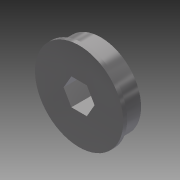
# Autodesk Inventor part: Hex Bearing 3-8 in (FR6ZZL-hex (am-0692))
Saved by Autodesk Inventor 2014 (Build 180170000, 170)
## iProperties
Created: 2014-01-12
Part Number: Hex Bearing 3-8 in (FR6ZZL-hex (am-0692))
Material: Steel, Alloy
Document SubType Name: Modeling
Designer: Michael
Density: 7.85 g/cm^3
Appearance: Semi-Polished
Author: Michael
Autodesk Inventor part; units mm, degrees
ref_plane "YZ Plane" through (0, 0, 0) normal (1, 0, 0) x (0, 1, 0)
ref_plane "XZ Plane" through (0, 0, 0) normal (0, 1, 0) x (-1, 0, 0)
ref_plane "XY Plane" through (0, 0, 0) normal (0, 0, 1) x (1, 0, 0)
sketch "Sketch1" plane through (0, 0, 0) normal (0, 0, 1) x (1, 0, 0)
  line L0 (2.7496, 4.7625) -> (5.4993, 0)
  line L1 (5.4993, 0) -> (2.7496, -4.7625)
  line L2 (2.7496, -4.7625) -> (-2.7496, -4.7625)
  line L3 (-2.7496, -4.7625) -> (-5.4993, 0)
  line L4 (-5.4993, 0) -> (-2.7496, 4.7625)
  line L5 (-2.7496, 4.7625) -> (2.7496, 4.7625)
  circle A0 centre (0, 0) radius 14.2875
  dimension "d0" = 9.525
  dimension "d1" = 28.575
  constraints: 12 end point, 2 coincident, 1 centre point, 1 horizontal, 13 other
  measures "d0" distance between parallel lines of L2 L5
  measures "d1" diameter of A0
extrude "Extrusion1" add sketch "Sketch1" along normal blind 6.35
sketch "Sketch2" plane through (0, 0, 6.35) normal (0, 0, 1) x (1, 0, 0)
  line L0 (5.4993, 0) -> (2.7496, -4.7625) projected
  line L1 (2.7496, -4.7625) -> (-2.7496, -4.7625) projected
  line L2 (-2.7496, -4.7625) -> (-5.4993, 0) projected
  line L3 (-5.4993, 0) -> (-2.7496, 4.7625) projected
  line L4 (-2.7496, 4.7625) -> (2.7496, 4.7625) projected
  line L5 (2.7496, 4.7625) -> (5.4993, 0) projected
  circle A0 centre (0, 0) radius 14.2875 projected
  circle A1 centre (0, 0) radius 15.6845
  dimension "d4" = 1.397
  constraints: 1 centre point, 1 coincident
  measures "d4" radial gap between concentric circles of A0 A1
extrude "Extrusion2" add sketch "Sketch2" along normal blind 1.397 contours A0 | A1
body "Solid1"
